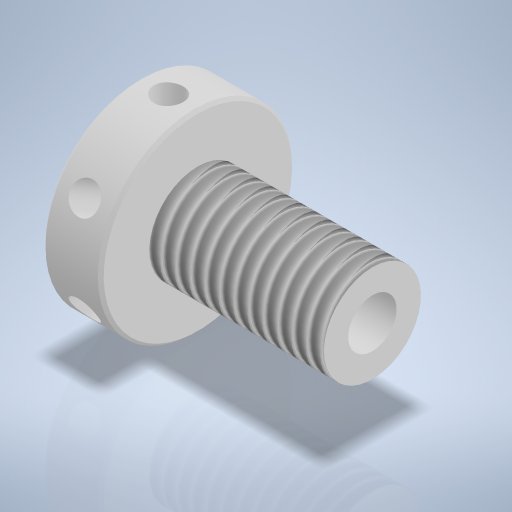
# Autodesk Inventor part: 1153
Saved by Autodesk Inventor 2024 (Build 280153000, 153)
## iProperties
Created: 2024-06-07
Part Number: 1153
Material: Generisch
Document SubType Name: Modeling
Designer: ffogue
Density: 1 g/cm^3
Appearance: Vorgabe
Author: ffogue
Autodesk Inventor part; units mm, degrees
ref_plane "YZ Plane" through (0, 0, 0) normal (1, 0, 0) x (0, 1, 0)
ref_plane "XZ Plane" through (0, 0, 0) normal (0, 1, 0) x (-1, 0, 0)
sketch "Skizze1" plane through (0, 0, 0) normal (0, 1, 0) x (-1, 0, 0)
  line L0 (0, 0) -> (0, 10)
  line L1 (0, 10) -> (-6, 10)
  line L2 (-6, 10) -> (-6, 5)
  line L3 (-6, 5) -> (-24, 5)
  line L4 (-24, 5) -> (-24, 0)
  line L5 (-24, 0) -> (0, 0)
  dimension "d0" = 20
  dimension "d1" = 10
  dimension "d2" = 6
  dimension "d3" = 18
  constraints: 12 end point, 5 perpendicular, 1 vertical
  measures "d0" diameter of L1 L5
  measures "d1" diameter of L3 L5
  measures "d2" distance between parallel lines of L0 L2
  measures "d3" distance between parallel lines of L4 L2
revolve "Umdrehung1" add sketch "Skizze1" angle 360 about axis through (24, 0, 0) along (-1, 0, 0)
sketch "Skizze2" plane through (24, 0, 0) normal (1, 0, 0) x (0, 0, -1)
  circle A0 centre (0, 0) radius 5 projected
  constraints: 1 coincident
hole "Bohrung1" at (24, 0, 0) direction (-1, 0, 0) diameter 5 depth 24
thread "Gewinde1" size "M10x1.5" class "6g" standard "ISO Metric profile" length 18
ref_plane "Arbeitsebene1" through (0, 0, 10) normal (0, 0, 1) x (1, 0, 0)
sketch "Skizze3" plane through (0, 0, 10) normal (0, 0, 1) x (1, 0, 0)
  line L0 (0, 10) -> (0, -10) projected
  point P0 (0, 0)
  point P1 (3, 0)
  point P2 (0, 0)
  dimension "d15" = 3
  constraints: 1 horizontal alignment, 1 midpoint
  measures "d15" distance from line of L0 point (3, 0)
hole "Bohrung2" at (3, 0, 10) direction (0, 0, -1) diameter 3 depth 6
pattern_circular "Runde Anordnung1" count 6 over 360 about axis through (3, 0, 0) along (-1, 0, 0) of "Bohrung2"
chamfer "Fasen1" distance 0.3 angle 45 2 edges at (0, 0, -10) (6, 0, -10)
